Simulation of affect of outside edge of lectures on a rotary bearing v8 (Autodesk Fusion 360 design; units mm, degrees)
Autodesk Fusion 360 part; units mm, degrees
sketch "Sketch1" plane through (0, 0, 0) normal (0, 0, 1) x (1, 0, 0)
  line L0 (-78.198, 0.5) -> (78.198, 0.5)
  line L1 (78.198, 0.5) -> (78.198, -0.5)
  line L2 (78.198, -0.5) -> (-78.198, -0.5)
  line L3 (-78.198, -0.5) -> (-78.198, 0.5)
  line L4 (-78.198, 0.5) -> (78.198, -0.5) construction
  line L5 (78.198, 0.5) -> (-78.198, -0.5) construction
  line L6 (-67.4715, -39.532) -> (-67.9715, -38.666)
  line L7 (-67.9715, -38.666) -> (67.9715, 38.666) construction
  line L8 (67.4715, 39.532) -> (67.9715, 38.666)
  line L9 (67.9715, 38.666) -> (-67.4715, -39.532)
  line L10 (-67.9715, -38.666) -> (67.4715, 39.532)
  line L11 (67.4715, 39.532) -> (-67.4715, -39.532) construction
  line L12 (-38.666, -67.9715) -> (-39.532, -67.4715)
  line L13 (-39.532, -67.4715) -> (39.532, 67.4715) construction
  line L14 (38.666, 67.9715) -> (39.532, 67.4715)
  line L15 (39.532, 67.4715) -> (-38.666, -67.9715)
  line L16 (-39.532, -67.4715) -> (38.666, 67.9715)
  line L17 (38.666, 67.9715) -> (-38.666, -67.9715) construction
  line L18 (0.5, -78.198) -> (-0.5, -78.198)
  line L19 (-0.5, -78.198) -> (0.5, 78.198) construction
  line L20 (-0.5, 78.198) -> (0.5, 78.198)
  line L21 (0.5, 78.198) -> (0.5, -78.198)
  line L22 (-0.5, -78.198) -> (-0.5, 78.198)
  line L23 (-0.5, 78.198) -> (0.5, -78.198) construction
  line L24 (39.532, -67.4715) -> (38.666, -67.9715)
  line L25 (38.666, -67.9715) -> (-38.666, 67.9715) construction
  line L26 (-39.532, 67.4715) -> (-38.666, 67.9715)
  line L27 (-38.666, 67.9715) -> (39.532, -67.4715)
  line L28 (38.666, -67.9715) -> (-39.532, 67.4715)
  line L29 (-39.532, 67.4715) -> (39.532, -67.4715) construction
  line L30 (67.9715, -38.666) -> (67.4715, -39.532)
  line L31 (67.4715, -39.532) -> (-67.4715, 39.532) construction
  line L32 (-67.9715, 38.666) -> (-67.4715, 39.532)
  line L33 (-67.4715, 39.532) -> (67.9715, -38.666)
  line L34 (67.4715, -39.532) -> (-67.9715, 38.666)
  line L35 (-67.9715, 38.666) -> (67.9715, -38.666) construction
  line L36 (78.198, 0.5) -> (78.198, -0.5)
  line L37 (78.198, -0.5) -> (-78.198, 0.5) construction
  line L38 (-78.198, -0.5) -> (-78.198, 0.5)
  line L39 (-78.198, 0.5) -> (78.198, 0.5)
  line L40 (78.198, -0.5) -> (-78.198, -0.5)
  line L41 (-78.198, -0.5) -> (78.198, 0.5) construction
  line L42 (67.4715, 39.532) -> (67.9715, 38.666)
  line L43 (67.9715, 38.666) -> (-67.9715, -38.666) construction
  line L44 (-67.4715, -39.532) -> (-67.9715, -38.666)
  line L45 (-67.9715, -38.666) -> (67.4715, 39.532)
  line L46 (67.9715, 38.666) -> (-67.4715, -39.532)
  line L47 (-67.4715, -39.532) -> (67.4715, 39.532) construction
  line L48 (38.666, 67.9715) -> (39.532, 67.4715)
  line L49 (39.532, 67.4715) -> (-39.532, -67.4715) construction
  line L50 (-38.666, -67.9715) -> (-39.532, -67.4715)
  line L51 (-39.532, -67.4715) -> (38.666, 67.9715)
  line L52 (39.532, 67.4715) -> (-38.666, -67.9715)
  line L53 (-38.666, -67.9715) -> (38.666, 67.9715) construction
  line L54 (-0.5, 78.198) -> (0.5, 78.198)
  line L55 (0.5, 78.198) -> (-0.5, -78.198) construction
  line L56 (0.5, -78.198) -> (-0.5, -78.198)
  line L57 (-0.5, -78.198) -> (-0.5, 78.198)
  line L58 (0.5, 78.198) -> (0.5, -78.198)
  line L59 (0.5, -78.198) -> (-0.5, 78.198) construction
  line L60 (-39.532, 67.4715) -> (-38.666, 67.9715)
  line L61 (-38.666, 67.9715) -> (38.666, -67.9715) construction
  line L62 (39.532, -67.4715) -> (38.666, -67.9715)
  line L63 (38.666, -67.9715) -> (-39.532, 67.4715)
  line L64 (-38.666, 67.9715) -> (39.532, -67.4715)
  line L65 (39.532, -67.4715) -> (-39.532, 67.4715) construction
  line L66 (-67.9715, 38.666) -> (-67.4715, 39.532)
  line L67 (-67.4715, 39.532) -> (67.4715, -39.532) construction
  line L68 (67.9715, -38.666) -> (67.4715, -39.532)
  line L69 (67.4715, -39.532) -> (-67.9715, 38.666)
  line L70 (-67.4715, 39.532) -> (67.9715, -38.666)
  line L71 (67.9715, -38.666) -> (-67.9715, 38.666) construction
  dimension "d1" = 1
  dimension "d3" = 360
  constraint horizontal L0
  constraint perpendicular L0 L1
  constraint parallel L0 L2
  constraint parallel L1 L3
  constraint coincident L4 origin
  constraint coincident L5 origin
  measures "d1" distance of L0.end L1.end
extrude "Extrude1" add sketch "Sketch1" along normal blind 132.557
